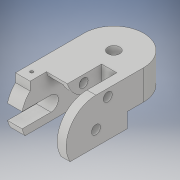
# Autodesk Inventor part: knuckle
Saved by Autodesk Inventor 2018 (Build 220112000, 112)
## iProperties
Created: 2017-10-01
Part Number: knuckle
Material: Generic
Document SubType Name: Modeling
Designer: Martin
Density: 1 g/cm^3
Appearance: Default
Author: Martin
Autodesk Inventor part; units mm, degrees
ref_plane "YZ Plane" through (0, 0, 0) normal (1, 0, 0) x (0, 1, 0)
ref_plane "XZ Plane" through (0, 0, 0) normal (0, 1, 0) x (-1, 0, 0)
ref_plane "XY Plane" through (0, 0, 0) normal (0, 0, 1) x (1, 0, 0)
sketch "Sketch1" plane through (0, 0, 0) normal (1, 0, 0) x (0, 1, 0)
  point P0 (0, 0)
sketch "Sketch2" plane through (0, 0, 0) normal (1, 0, 0) x (0, 1, 0)
  arc A0 (10, 0) -> (-10, 0) centre (0, 0) ccw
  circle A1 centre (0, 0) radius 1.5
  line L0 (10, 0) -> (-10, 0)
  line L1 (-10, 0) -> (-10, -16)
  line L2 (0, -26) -> (10, -26)
  line L3 (10, -26) -> (10, 0)
  line L4 (0, -26) -> (0, -16)
  line L5 (0, -16) -> (-10, -16)
  dimension "d1" = 3
  constraints: 12 end point, 2 centre point, 2 coincident, 2 parallel, 2 point on circle, 1 horizontal, 1 perpendicular
  measures "d1" diameter of A1
extrude "Extrusion1" add sketch "Sketch2" along normal blind 20
sketch "Sketch3" plane through (0, 10, 0) normal (0, 1, 0) x (1, 0, 0)
  line L0 (0, 26) -> (20, 26) projected
  line L1 (0, 16) -> (20, 16) projected
  arc A0 (20, 16) -> (0, 16) centre (10, 16) ccw
  line L2 (21.9475, 16) -> (-2.9161, 16)
  line L3 (-2.9161, 16) -> (-2.9161, 27.442)
  line L4 (-2.9161, 27.442) -> (21.9475, 27.442)
  line L5 (21.9475, 27.442) -> (21.9475, 16)
  point P0 (0, 0)
  constraints: 10 end point, 2 parallel, 2 point on circle, 1 centre point, 1 horizontal, 1 perpendicular, 1 tangent
extrude "Extrusion2" cut sketch "Sketch3" against normal blind 20 contours L2 L3 L4 L5 A0
sketch "Sketch5" plane through (0, 10, 0) normal (0, 1, 0) x (1, 0, 0)
  line L0 (0, -10) -> (20, -10) projected
  line L1 (0, -10) -> (4.9, -10)
  line L2 (4.9, -10) -> (4.9, 10)
  line L3 (4.9, 10) -> (17, 10)
  line L4 (17, 10) -> (17, -10)
  line L5 (17, -10) -> (4.9, -10)
  point P0 (0, 0)
  dimension "d10" = 4.9
  dimension "d11" = 20
  dimension "d12" = 12.1
  constraints: 10 end point, 3 perpendicular, 3 point on line, 1 collinear
  measures "d10" distance of L1.start L1.end
  measures "d11" distance of L1.end L2.end
  measures "d12" distance of L2.end L3.end
extrude "Extrusion3" cut sketch "Sketch5" against normal blind 20
sketch "Sketch6" plane through (0, 0, 0) normal (-1, 0, 0) x (0, 0, 1)
  arc A0 (0, 2.5) -> (0, -2.5) centre (0, 0) ccw
  line L0 (0, 2.5) -> (12.401, 2.5)
  line L1 (12.401, 2.5) -> (12.401, -2.5)
  line L2 (12.401, -2.5) -> (0, -2.5)
  dimension "d15" = 5
  constraints: 6 end point, 2 point on circle, 1 centre point, 1 coincident, 1 horizontal, 1 parallel, 1 perpendicular
  measures "d15" diameter of A0
extrude "Extrusion4" cut sketch "Sketch6" against normal blind 5
sketch "Sketch7" plane through (0, 0, 0) normal (-1, 0, 0) x (0, 0, 1)
  line L0 (-16, -10) -> (12.5782, -10)
  line L1 (12.5782, -10) -> (12.5782, -5)
  line L2 (12.5782, -5) -> (-16, -5)
  line L3 (-16, -5) -> (-16, -10)
  point P0 (0, 0)
  dimension "d18" = 5
  constraints: 8 end point, 2 parallel, 1 horizontal, 1 perpendicular
  measures "d18" distance of L1.end L0.end
extrude "Extrusion5" cut sketch "Sketch7" against normal through all
sketch "Sketch8" plane through (0, 10, 0) normal (0, 1, 0) x (1, 0, 0)
  line L0 (0, 16) -> (20, 16) projected
  circle A0 centre (10, 16) radius 2
  point P0 (0, 0)
  dimension "d21" = 4
  constraints: 1 centre point, 1 midpoint
  measures "d21" diameter of A0
extrude "Extrusion6" cut sketch "Sketch8" against normal through all
sketch "Sketch9" plane through (0, -5, -16) normal (0, -1, 0) x (1, 0, 0)
  line L0 (0, 0) -> (8, 0) projected
  line L1 (12, 0) -> (20, 0) projected
  line L2 (8, 0) -> (12, 0)
  circle A0 centre (10, 0) radius 4.5
  point P0 (0, 16)
  dimension "d24" = 9
  constraints: 2 end point, 1 centre point, 1 collinear, 1 midpoint
  measures "d24" diameter of A0
extrude "Extrusion7" cut sketch "Sketch9" against normal blind 10
sketch "Sketch12" plane through (0, -5, -16) normal (0, -1, 0) x (1, 0, 0)
  arc A0 (14.5, 0) -> (5.5, 0) centre (10, 0) ccw projected
  line L0 (4.9, 6) -> (17, 6) projected
  line L1 (9, 6) -> (9, 4.2062)
  line L2 (11, 6) -> (11, 4.2062)
  line L3 (9, 4.2062) -> (11, 4.2062)
  line L4 (9, 6) -> (11, 6)
  point P0 (0, 16)
  constraints: 8 end point, 1 collinear, 1 perpendicular
extrude "Extrusion8" cut sketch "Sketch12" against normal blind 4
sketch "Sketch13" plane through (0, -5, -16) normal (0, -1, 0) x (1, 0, 0)
  arc A0 (5.5, 0) -> (-5.5, 0) centre (0, 0) ccw
  arc A1 (25.5, 0) -> (14.5, 0) centre (20, 0) ccw
  line L0 (26.0588, 0) -> (26.0588, -15.4765)
  line L1 (26.0588, -15.4765) -> (-5.5, -15.4765)
  line L2 (-5.5, -15.4765) -> (-5.5, 0)
  line L3 (5.5, 0) -> (14.5, 0)
  line L4 (25.5, 0) -> (26.0588, 0)
  point P0 (0, 16)
  dimension "d33" = 11
  dimension "d34" = 11
  constraints: 10 end point, 4 point on circle, 3 parallel, 2 centre point, 2 horizontal, 2 perpendicular
  measures "d33" diameter of A0
  measures "d34" diameter of A1
extrude "Extrusion9" cut sketch "Sketch13" against normal blind 5
sketch "Sketch14" plane through (20, 0, 0) normal (1, 0, 0) x (0, 0, -1)
  circle A0 centre (3.94, 7.53) radius 1.5
  point P0 (0, 0)
  point P1 (0, 10)
  dimension "d39" = 3
  constraints: 1 centre point
  measures "d39" diameter of A0
extrude "Extrusion10" cut sketch "Sketch14" against normal blind 5
sketch "Sketch15" plane through (20, 0, 0) normal (1, 0, 0) x (0, 0, -1)
  circle A0 centre (0, 0) radius 1.5
  dimension "d43" = 3
  constraints: 1 centre point, 1 coincident
  measures "d43" diameter of A0
extrude "Extrusion11" cut sketch "Sketch15" against normal blind 5
sketch "Sketch16" plane through (4.9, 10, 0) normal (1, 0, 0) x (0, 0, -1)
  line L0 (0, 0) -> (-1.5, 0)
  line L1 (-1.5, 0) -> (-1.5, -1.5)
  line L2 (-1.5, -1.5) -> (11.5, -1.5)
  line L3 (11.5, -1.5) -> (11.5, 0)
  line L4 (16, 0) -> (0, 0) projected
  line L5 (11.5, 0) -> (0, 0)
  point P0 (0, -10)
  dimension "d46" = 1.5
  dimension "d47" = 1.5
  dimension "d48" = 13
  constraints: 10 end point, 3 perpendicular, 1 collinear, 1 horizontal, 1 point on line
  measures "d46" distance of L0.start L0.end
  measures "d47" distance of L0.end L1.end
  measures "d48" distance of L1.end L2.end
extrude "Extrusion12" add sketch "Sketch16" along normal blind 7
sketch "Sketch17" plane through (0, 0, 0) normal (-1, 0, 0) x (0, 0, 1)
  line L0 (9.6825, 2.5) -> (0, 2.5) projected
  line L1 (0, 2.5) -> (7, 2.5)
  line L2 (7, 2.5) -> (7, 10)
  line L3 (7, 10) -> (0, 10)
  line L4 (0, 10) -> (0, 2.5)
  point P0 (0, 0)
  dimension "d51" = 7
  dimension "d52" = 7.5
  constraints: 8 end point, 2 parallel, 1 horizontal, 1 perpendicular
  measures "d51" distance of L3.end L2.end
  measures "d52" distance of L2.end L1.end
extrude "Extrusion13" add sketch "Sketch17" against normal blind 4.9
sketch "Sketch18" plane through (10, 10, -16) normal (0, 1, 0) x (1, 0, 0)
  circle A0 centre (-7.55, -20) radius 0.5
  line L0 (-5.1, -23) -> (-10, -23) projected
  line L1 (-7.55, -23) -> (-7.55, -20)
  point P0 (-10, -16)
  dimension "d55" = 1
  dimension "d58" = 3
  constraints: 2 end point, 1 centre point, 1 midpoint, 1 perpendicular
  measures "d55" diameter of A0
  measures "d58" distance of L1.start L1.end
extrude "Extrusion14" cut sketch "Sketch18" against normal up to next
sketch "Sketch19" plane through (17, -5, -10) normal (0, 0, 1) x (1, 0, 0)
  line L0 (-5.1, 13.5) -> (-12.1, 13.5) projected
  line L1 (-5.1, 13.5) -> (-5.1, 8.65)
  line L2 (-5.1, 8.65) -> (-7.1, 8.65)
  line L3 (-7.1, 8.65) -> (-7.1, 13.5)
  line L4 (-5.1, 15) -> (-5.1, 13.5) projected
  line L5 (-7.1, 13.5) -> (-5.1, 13.5)
  point P0 (-17, 5)
  dimension "d59" = 4.85
  dimension "d60" = 2
  constraints: 8 end point, 2 perpendicular, 1 horizontal, 1 point on line, 1 vertical
  measures "d59" distance of L0.start L1.end
  measures "d60" distance of L1.end L2.end
extrude "Extrusion15" add sketch "Sketch19" along normal blind 12
sketch "Sketch20" plane through (11.9, 10, 0) normal (1, 0, 0) x (0, 0, -1)
  circle A0 centre (3.94, -2.47) radius 1.5 projected
  circle A1 centre (3.94, -2.47) radius 1.5
  point P0 (0, -10)
  constraints: 1 centre point, 1 coincident
extrude "Extrusion16" cut sketch "Sketch20" against normal blind 2
sketch "Sketch21" plane through (11.9, 10, 0) normal (1, 0, 0) x (0, 0, -1)
  line L0 (-7.3238, -1.5) -> (-7.3238, -7.2177)
  line L1 (-7.3238, -7.2177) -> (-1.5, -7.2177)
  line L2 (-1.5, -7.2177) -> (4.1962, -7.2177)
  line L3 (10, -6.35) -> (-2, -6.35) projected
  line L4 (-1.5, 0) -> (-1.5, -1.5) projected
  line L5 (-1.5, 0) -> (-7.3238, 0)
  line L6 (-7.3238, 0) -> (-7.3238, -1.5)
  line L7 (-1.5, -0.1522) -> (-1.5, 0)
  line L8 (4.1962, -7.2177) -> (6.1782, -7.2177)
  line L9 (6.1782, -7.2177) -> (6.1782, -6.35)
  arc A0 (-1.5, 0) -> (6.141, -6.35) centre (6.8954, 2.33) ccw
  point P0 (0, -10)
  point P1 (4.1962, -6.35)
  point P2 (3.0513, -6.35)
  constraints: 16 end point, 3 point on line, 2 point on circle, 1 centre point, 1 horizontal, 1 parallel, 1 perpendicular
extrude "Extrusion17" cut sketch "Sketch21" against normal blind 7
body "Solid1"
